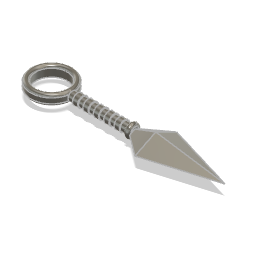
kunai v1 (Autodesk Fusion 360 design; units mm, degrees)
Autodesk Fusion 360 part; units mm, degrees
sketch "Sketch1" plane through (0, 0, 0) normal (1, 0, 0) x (0, 0, -1)
  line L0 (60, 30) -> (-60, 30)
  line L1 (-60, 30) -> (-60, -30)
  line L2 (-60, -30) -> (60, -30)
  line L3 (60, -30) -> (60, 30)
  line L4 (60, 30) -> (-60, -30) construction
  line L5 (-60, 30) -> (60, -30) construction
  line L6 (0, 30) -> (-60, 0)
  line L7 (-60, 0) -> (0, -30)
  line L8 (0, 30) -> (60, 0)
  line L9 (60, 0) -> (0, -30)
  dimension "d1" = 120
  constraint horizontal L0
  constraint perpendicular L0 L1
  constraint parallel L0 L2
  constraint parallel L1 L3
  constraint coincident L4 origin
  constraint coincident L5 origin
  constraint midpoint L0 L6.start
  constraint midpoint L1 L6.end
  constraint midpoint L2 L7.end
  measures "d1" distance of L1.end L2.end
ref_plane "WorkPlane1" through (200, 0, 0) normal (1, 0, 0) x (0, 0, -1)
sketch "Sketch2" plane through (0, 0, 0) normal (1, 0, 0) x (0, 0, -1)
  point P0 (209.5412, -206.1772)
sketch "Sketch3" plane through (200, 0, 0) normal (1, 0, 0) x (0, 0, -1)
loft "Loft1" add profiles "Sketch1" section 1 contours L6 L7 L8 L9 section 2 point at (200, 0, 0) makes body 1
sketch "Sketch4" plane through (0, 0, 0) normal (-1, 0, 0) x (0, 0, 1)
  line L0 (60, 0) -> (0, 30)
  line L1 (0, 30) -> (-60, 0)
  line L2 (-60, 0) -> (0, -30)
  line L3 (0, -30) -> (60, 0)
ref_plane "WorkPlane2" through (-60, 0, 0) normal (-1, 0, 0) x (0, 0, 1)
sketch "Sketch5" plane through (-60, 0, 0) normal (-1, 0, 0) x (0, 0, 1)
  line L0 (15.3234, 7.4489) -> (-15.3234, 7.4489)
  line L1 (-15.3234, 7.4489) -> (-15.3234, -7.4489)
  line L2 (-15.3234, -7.4489) -> (15.3234, -7.4489)
  line L3 (15.3234, -7.4489) -> (15.3234, 7.4489)
  line L4 (15.3234, 7.4489) -> (-15.3234, -7.4489) construction
  line L5 (-15.3234, 7.4489) -> (15.3234, -7.4489) construction
  line L6 (0, 7.4489) -> (-15.3234, 0)
  line L7 (-15.3234, 0) -> (0, -7.4489)
  line L8 (0, 7.4489) -> (15.3234, 0)
  line L9 (15.3234, 0) -> (0, -7.4489)
  constraint horizontal L0
  constraint perpendicular L0 L1
  constraint parallel L0 L2
  constraint parallel L1 L3
  constraint coincident L4 origin
  constraint coincident L5 origin
  constraint midpoint L0 L6.start
  constraint midpoint L1 L6.end
  constraint midpoint L2 L7.end
  constraint midpoint L3 L8.end
loft "Loft2" add profiles "Sketch5", "Sketch4" section 1 contours L6 L7 L8 L9 section 2 bodies 1
cylinder "CylinderPrimitive1" add diameter 40 height 15 placed x (0, 0, 1) y (0, 1, 0) z (-1, 0, 0) at (-60, 0, 0) bodies 1
fillet "Fillet1" radius 7.5 1 edges at (-60, 7.2323, -18.6465) on bodies 1
fillet "Fillet2" radius 7.5 1 edges at (-75, -7.2323, -18.6465) on bodies 1
cylinder "CylinderPrimitive2" add diameter 25 height 15 placed x (0, 0, 1) y (0, 1, 0) z (-1, 0, 0) at (-75, 0, 0) separate body makes body 2
cylinder "CylinderPrimitive3" add diameter 30 height 15 placed x (0, 0, 1) y (0, 1, 0) z (-1, 0, 0) at (-90, 0, 0) separate body makes body 3
pattern_linear "R-Pattern1" count 6 spacing 30 along (-1, 0, 0) of bodies 3 2 makes body 4 at (-110, -1.2446, 12.4379) makes body 5 at (-140, -1.2446, 12.4379) makes body 6 at (-170, -1.2446, 12.4379) makes body 7 at (-200, -1.2446, 12.4379) makes body 8 at (-230, -1.2446, 12.4379) makes body 9 at (-125, -1.4935, 14.9255) makes body 10 at (-155, -1.4935, 14.9255) makes body 11 at (-185, -1.4935, 14.9255) makes body 12 at (-215, -1.4935, 14.9255) makes body 13 at (-245, -1.4935, 14.9255)
sketch "Sketch9" plane through (0, 0, 0) normal (0, 1, 0) x (1, 0, 0)
  circle A0 centre (-300, 0) radius 60
  circle A1 centre (-300, 0) radius 45
  dimension "d18" = 90
  constraint concentric A0 A1
  measures "d18" diameter of A1
extrude "Extrude1" add sketch "Sketch9" along normal mid plane 30 separate body makes body 14
fillet "Fillet3" radius 7.5 1 edges at (-355.9396, 15, 21.6969) 1 faces at (-245.2234, 15, 2.9808) on bodies 14
fillet "Fillet4" radius 7.5 1 edges at (-355.9396, -15, -21.6969) on bodies 14
fillet "Fillet5" radius 7.5 1 edges at (-240, 5.4242, -13.9849) on bodies 13
fillet "Fillet6" radius 7.5 1 edges at (-255, -5.4242, -13.9849) on bodies 13
sketch "Sketch10" plane through (0, 0, 0) normal (1, 0, 0) x (0, 0, -1)
